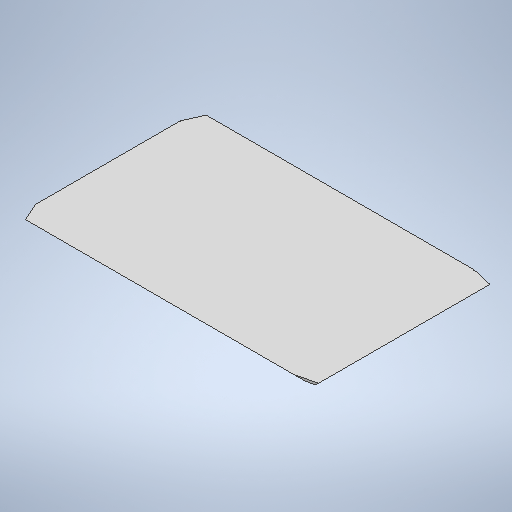
# Autodesk Inventor part: Part3
Saved by Autodesk Inventor 2025.2 (Build 292293000, 293)
## iProperties
Created: 2025-06-06
Part Number: Part3
Material: Generic
Document SubType Name: Sheet Metal
Designer: ziyuz
Density: 1 g/cm^3
Sheet Metal Rule: Default_mm
Appearance: Default
Author: ziyuz
Autodesk Inventor part; units mm, degrees
ref_plane "YZ Plane" through (0, 0, 0) normal (1, 0, 0) x (0, 1, 0)
ref_plane "XZ Plane" through (0, 0, 0) normal (0, 1, 0) x (-1, 0, 0)
ref_plane "XY Plane" through (0, 0, 0) normal (0, 0, 1) x (1, 0, 0)
sketch "Sketch1" plane through (0, 0, 0) normal (0, 1, 0) x (-1, 0, 0)
  line L0 (0, -21.606) -> (2.93, -21.606) construction
  line L1 (-2.6765, -22.7982) -> (-42.6765, -22.7982)
  line L2 (-2.6765, -22.7982) -> (37.3235, -22.7982) construction
  line L3 (-42.6765, -22.7982) -> (-45.7255, -22.0954)
  line L4 (-42.6765, -22.7982) -> (-39.5475, -22.7982) construction
  line L5 (-45.7255, -22.0954) -> (-45.7255, 3.4986)
  line L6 (-42.6765, -22.7982) -> (-42.6765, 4.2018)
  line L7 (-45.7255, 3.4986) -> (-42.6765, 4.2018)
  line L8 (-42.6765, 4.2018) -> (-2.6765, 4.2018)
  line L9 (-42.6765, 4.2018) -> (-2.6765, 4.2018) construction
  line L10 (-2.6765, 4.2018) -> (-1.4749, 1.5043)
  line L11 (-2.6765, 4.2018) -> (0.2765, 4.2018) construction
  line L12 (-1.4749, 1.5043) -> (-1.4749, -20.1017)
  line L13 (-1.4749, -20.1017) -> (-2.6765, -22.7982)
  point P0 (0, 0)
  dimension "d0" = 21.606
  dimension "d1" = 2.93
  dimension "d3" = 40
  dimension "d4" = 180
  dimension "d5" = 3.129
  dimension "d6" = 167.02
  dimension "d7" = 25.594
  dimension "d8" = 27
  dimension "d9" = 40
  dimension "d10" = 0
  dimension "d11" = 2.953
  dimension "d12" = 65.99
  dimension "d13" = 21.606
  constraints: 28 end point, 7 horizontal, 4 equal length, 3 vertical
  measures "d0" distance of point (0, 0) L0.start
  measures "d1" distance of L0.start L1.start
  measures "d3" distance of L1.start L1.end
  measures "d4" angle of L1 L2
  measures "d5" distance of L1.end L3.end
  measures "d6" angle of L4 L3
  measures "d7" distance of L3.end L5.end
  measures "d8" distance of L1.end L6.end
  measures "d9" distance of L6.end L8.end
  measures "d10" distance between parallel lines of L8 L9
  measures "d11" distance of L9.end L10.end
  measures "d12" angle of L10 L11
  measures "d13" distance of L10.end L12.end
extrude "Extrusion1" add sketch "Sketch1" along normal blind 2
chamfer "Chamfer1" distance 2 angle 45 8 edges at (22.6765, 0, 4.2018) (2.0757, 0, 2.853) (1.4749, 0, -9.2987) (2.0757, 0, -21.45) (22.6765, 0, -22.7982) (44.201, 0, -22.4468) (45.7255, 0, -9.2984) (44.201, 0, 3.8502)
equation "\"BendRadius\" = Thickness"
equation "\"BendReliefWidth\" = Thickness"
equation "\"BendReliefDepth\" = 0.5 * Thickness"
equation "\"CornerReliefSize\" = 4 * Thickness"
equation "\"MinimumRemnant\" = 2 * Thickness"
equation "\"TransitionRadius\" = BendRadius"
equation "\"JacobiRadiusSize\" = BendRadius"
equation "\"GapSize\" = Thickness"
equation "\"Thickness\" = 0.5"
body "Solid1"
